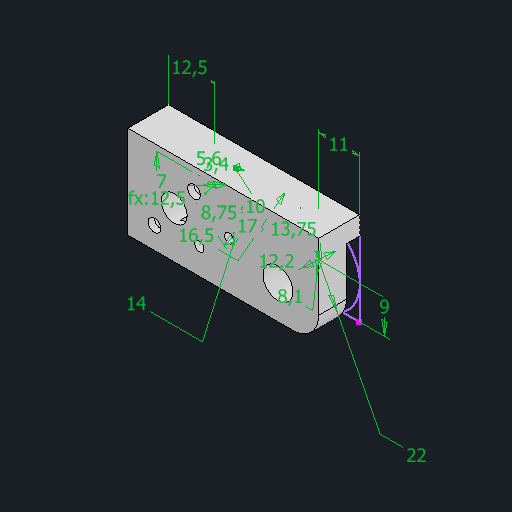
# Autodesk Inventor part: MocowaniePrzekladni_CPY
Saved by Autodesk Inventor 2023 (Build 270158000, 158)
## iProperties
Created: 2024-02-25
Part Number: MocowaniePrzekladni_CPY
Material: Generic
Document SubType Name: Modeling
Designer: Michał
Density: 1 g/cm^3
Appearance: Default
Author: Michał
Autodesk Inventor part; units mm, degrees
ref_plane "YZ Plane" through (0, 0, 0) normal (1, 0, 0) x (0, 1, 0)
ref_plane "XZ Plane" through (0, 0, 0) normal (0, 1, 0) x (-1, 0, 0)
ref_plane "XY Plane" through (0, 0, 0) normal (0, 0, 1) x (1, 0, 0)
sketch "Sketch1" plane through (0, 0, 0) normal (0, 0, 1) x (1, 0, 0)
  line L0 (45, 0) -> (-6.5, 0) projected
  line L1 (-6.5, 0) -> (-6.5, 25) projected
  line L2 (45, 25) -> (-6.5, 25) projected
  line L3 (45, 0) -> (45, 25) projected
  circle A0 centre (12.8053, 7) radius 1.25 projected
  circle A1 centre (20.8333, 12.9625) radius 1.25 projected
  circle A2 centre (34, 9) radius 3 projected
extrude "Bryla" add sketch "Sketch1" along normal blind 11 contours L0 L1 L2 L3 | A0 | A1 | A2
sketch "Sketch3" plane through (0, 0, 0) normal (0, 0, -1) x (-1, 0, 0)
  circle A0 centre (-6, 12.5) radius 3.5
  circle A1 centre (-12.8053, 7) radius 7
  circle A2 centre (-20.8333, 12.9625) radius 8.25
  circle A3 centre (-34, 9) radius 11
  circle A4 centre (-34, 9) radius 4.05
  circle A5 centre (-34, 9) radius 6.1
  line L0 (-6, 12.5) -> (-12.8053, 7) construction
  line L1 (-12.8053, 7) -> (-20.8333, 12.9625) construction
  line L2 (-20.8333, 12.9625) -> (-34, 9) construction
  line L3 (-11.3429, 19.1109) -> (-0.6571, 5.8891) construction
  circle A6 centre (-0.6571, 5.8891) radius 1.7
  circle A7 centre (-11.3429, 19.1109) radius 1.7
  circle A8 centre (-11.3429, 19.1109) radius 2.8
  circle A9 centre (-0.6571, 5.8891) radius 2.8
  line L4 (6.5, 25) -> (6.5, 0) construction
  line L5 (6.5, 0) -> (-45, 0) construction
  line L6 (-45, 0) -> (-45, 25) construction
  line L7 (-34, 20) -> (-45, 20)
  line L8 (-45, 20) -> (-45, 0)
  line L9 (6.5, 0) -> (-45, 0) projected
  line L10 (-40.3246, 0) -> (-45, 0)
  line L11 (-27.6754, 0) -> (-23, 0)
  line L12 (-23, 0) -> (-23, 9)
  line L13 (-19.8053, 7) -> (-19.8053, 0)
  line L14 (-5.8053, 7) -> (-5.8053, 0)
  line L15 (-23, 0) -> (-19.8053, 0)
  line L16 (-29.0833, 12.9625) -> (-29.0833, 0)
  line L17 (-29.0833, 0) -> (-27.6754, 0)
  point P0 (-27.9066, 8.7162)
  point P1 (-29.0753, 12.5997)
  point P2 (-19.4597, 4.8276)
  point P3 (-22.8938, 18.8508)
  point P4 (-23.6713, 5.216)
  point P5 (-25.7685, 19.5736)
  point P6 (-12.819, 14.9204)
  point P7 (-27.4753, 17.856)
  point P8 (-20.5208, 12.676)
  point P9 (-12.6486, 13.9982)
  point P10 (-18.4098, 11.1941)
  point P11 (-8.5508, 12.5587)
  point P12 (-1.1315, 7.6691)
  point P13 (-9.5, 12.5)
  point P14 (-2.6315, 11.5495)
  point P15 (-9.4412, 13.1386)
  point P16 (-6.1553, 9.4162)
  point P17 (-8.5736, 18.697)
  point P18 (-9.3, 21.0258)
  point P19 (-6.0975, 9.0014)
  point P20 (-27.6754, 0)
  point P21 (-12.8053, 0)
  point P22 (-19.8053, 4.7768)
  point P23 (-23, 5.0021)
  dimension "d20" = 7
  dimension "d21" = 14
  dimension "d22" = 16.5
  dimension "d23" = 22
  dimension "d24" = 12.2
  dimension "d25" = 8.1
  dimension "d26" = 8.75
  dimension "d27" = 10
  dimension "d28" = 13.75
  dimension "d59" = 5.6
  dimension "d60" = 3.4
  dimension "d61" = 17
  dimension "d65" = 12.5
  dimension "d66" = 12.5
  dimension "d68" = 11
  dimension "d69" = 9
  constraints: 28 end point, 16 point on circle, 9 centre point, 7 coincident, 6 tangent, 5 point on line, 4 vertical, 3 horizontal, 2 collinear, 2 perpendicular, 1 equal radius, 1 midpoint, 2 other
  measures "d20" diameter of A0
  measures "d21" diameter of A1
  measures "d22" diameter of A2
  measures "d23" diameter of A3
  measures "d24" diameter of A5
  measures "d25" diameter of A4
  measures "d26" distance of L0.start L0.end
  measures "d27" distance of L0.end L1.end
  measures "d28" distance of L1.end L2.end
  measures "d59" diameter of A8
  measures "d60" diameter of A7
  measures "d61" distance of L3.start L3.end
  measures "d65" distance from line of L4 L0.start
  measures "d66" distance from line of L5 L0.start
  measures "d68" distance from line of L6 A3.centre
  measures "d69" distance from line of L5 A3.centre
extrude "Przelot" cut sketch "Sketch3" against normal through all contours A0 A1 | A1 A0 | A4 | A6 | A7
extrude "kolo3" cut sketch "Sketch3" against normal blind 3.5 contours A1 A0 | A3 A2 A5 | A2 L16 A5 L9 A3 | L13 L9 L12 A2 | A2 A5 L16 | L12 A2 A3 | A3 L8 L7 | L12 L9 A3 A2 | A5 A2 | A2 A5 L16 | L16 A5 | A3 L9 L16 A5 A2 | A3 L9 L8 | A3 L9 | A4 picked at (-7.468, 10.5481)
extrude "kolo1" cut sketch "Sketch3" against normal blind 9.3 contours A0 A1 | A1 A0 | A0 A1 A2 | A2 A1 | L14 L9 A1 | A1 A2 L13 | L9 L13 A2 A1
extrude "kolo2" cut sketch "Sketch3" against normal blind 5.7 contours A2 A1 | A1 L13 A2 L12 A3 | A1 A2 L13 | A3 A2 A5 | L12 A2 A3 | A5 A2
hole "osieMale" at (20.8333, 12.9625, 0) at (12.8053, 7, 0) direction (0, 0, 1) diameter 2.5 end through all
extrude "kolnierzLozyska" cut sketch "Sketch3" against normal blind 1 from surface at -3.5 contours A2 A5 L16 | L16 A5 picked at (-28.8319, 8.8586)
extrude "lbySrob" cut sketch "Sketch3" against normal up to surface (9.3 mm away) contours A6 | A7 | A8 | A9
sketch "Sketch5" plane through (-6.5, 0, 11) normal (0, -1, 0) x (1, 0, 0)
  line L0 (0, -11) -> (0, 0) construction
  point P0 (6.5, -11)
  point P1 (3, -5.5)
  point P2 (0, -5.5)
  dimension "d71" = 3
  constraints: 1 horizontal alignment, 1 midpoint
  measures "d71" distance from line of L0 point (3, -5.5)
hole "Hole3" at (-3.5, 0, 5.5) direction (0, 1, 0) diameter 2.459 depth 6 tip angle 118 thread size "M3x0.5" class "6H" standard "ISO Metric profile"
fillet "Fillet1" radius 7 1 edges at (45, 0, 7.25)
body "Solid1"
